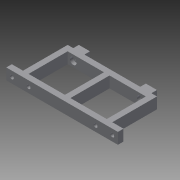
# Autodesk Inventor part: brush holder stand v5
Saved by Autodesk Inventor 2013 SP2 (Build 170200200, 200)
## iProperties
Created: 2018-02-20
Part Number: brush holder stand v5
Material: Generic
Document SubType Name: Modeling
Designer: hdv
Density: 1 g/cm^3
Author: hdv
Autodesk Inventor part; units mm, degrees
ref_plane "YZ Plane" through (0, 0, 0) normal (1, 0, 0) x (0, 1, 0)
ref_plane "XZ Plane" through (0, 0, 0) normal (0, 1, 0) x (-1, 0, 0)
ref_plane "XY Plane" through (0, 0, 0) normal (0, 0, 1) x (1, 0, 0)
sketch "Sketch1" plane through (0, 0, 0) normal (0, 0, 1) x (1, 0, 0)
  line L0 (0, 0) -> (80, 0)
  line L1 (80, 0) -> (80, 50)
  line L2 (80, 50) -> (0, 50)
  line L3 (0, 50) -> (0, 0)
  line L4 (15, 50) -> (65, 50)
  line L5 (65, 50) -> (65, 45)
  line L6 (65, 45) -> (15, 45)
  line L7 (15, 45) -> (15, 50)
  line L8 (5, 40) -> (75, 40)
  line L9 (75, 40) -> (75, 5)
  line L10 (75, 5) -> (5, 5)
  line L11 (5, 5) -> (5, 40)
  line L12 (-10, 0) -> (90, 0)
  line L13 (90, 0) -> (90, 5)
  line L14 (90, 5) -> (-10, 5)
  line L15 (-10, 5) -> (-10, 0)
  line L16 (0, 50) -> (5, 50)
  line L17 (5, 50) -> (5, 45)
  line L18 (5, 45) -> (0, 45)
  line L19 (0, 45) -> (0, 50)
  line L20 (80, 50) -> (75, 50)
  line L21 (75, 50) -> (75, 45)
  line L22 (75, 45) -> (80, 45)
  line L23 (80, 45) -> (80, 50)
  line L24 (37.5, 40) -> (42.5, 40)
  line L25 (42.5, 40) -> (42.5, 5)
  line L26 (42.5, 5) -> (37.5, 5)
  line L27 (37.5, 5) -> (37.5, 40)
  point P0 (40, 50)
  point P1 (40, 5)
  point P2 (40, 0)
  point P3 (40, 40)
  dimension "d0" = 80
  dimension "d1" = 50
  dimension "d2" = 50
  dimension "d3" = 70
  dimension "d4" = 100
  dimension "d5" = 5
  dimension "d6" = 5
  dimension "d7" = 5
  dimension "d10" = 5
  dimension "d11" = 5
  dimension "d12" = 5
  constraints: 56 end point, 14 parallel, 8 midpoint, 7 horizontal, 7 perpendicular, 4 point on line, 2 collinear
  measures "d0" distance of L2.end L1.end
  measures "d1" distance of L1.end L0.end
  measures "d2" distance of L5.end L6.end
  measures "d3" distance of L8.start L8.end
  measures "d4" distance of L12.start L12.end
  measures "d5" distance of L6.end L4.start
  measures "d6" distance of L14.end L12.start
  measures "d7" distance between parallel lines of L6 L8
  measures "d10" distance of L17.end L18.end
  measures "d11" distance of L22.end L21.end
  measures "d12" distance between parallel lines of L25 L27
extrude "Extrusion1" add sketch "Sketch1" along normal blind 10 contours L3 L14 L10 L1 L0 | L12 L15 L14 L3 | L1 L14 L13 L12 | L3 L18 L17 L2 L7 L6 L5 L21 L22 L1 L14 L9 L8 L11 | L27 L8 L25 L10
sketch "Sketch2" plane through (5, 50, 0) normal (0, 1, 0) x (1, 0, 0)
  line L0 (10, 0) -> (0, 0) projected
  circle A0 centre (5, -5) radius 1.7
  circle A1 centre (-10, -5) radius 1.7
  circle A2 centre (65, -5) radius 1.7
  circle A3 centre (80, -5) radius 1.7
  line L1 (70, -10) -> (70, 0) projected
  line L2 (70, 0) -> (60, 0) projected
  line L3 (85, 0) -> (75, 0) projected
  line L4 (-5, 0) -> (-15, 0) projected
  point P0 (70, -5)
  point P1 (5, 0)
  point P2 (65, 0)
  point P3 (80, 0)
  point P4 (-10, 0)
  dimension "d13" = 3.4
  constraints: 5 midpoint, 4 centre point, 4 horizontal alignment, 4 vertical alignment, 3 equal radius
  measures "d13" diameter of A0
extrude "Extrusion2" cut sketch "Sketch2" against normal through all
sketch "Sketch3" plane through (5, 40, 10) normal (0, -1, 0) x (1, 0, 0)
  circle A0 centre (5, -5) radius 1.7 projected
  circle A1 centre (5, -5) radius 3
  circle A2 centre (65, -5) radius 1.7 projected
  circle A3 centre (65, -5) radius 3
  point P0 (-5, -10)
  dimension "d17" = 6
  dimension "d18" = 6
  constraints: 2 centre point, 2 coincident
  measures "d17" diameter of A1
  measures "d18" diameter of A3
extrude "Extrusion3" cut sketch "Sketch3" against normal blind 3
body "Solid1"
